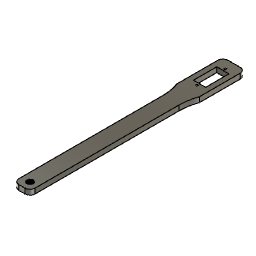
SOAR_Arm_Long-v2 (Autodesk Fusion 360 design; units mm, degrees)
Autodesk Fusion 360 part; units mm, degrees
sketch "Sketch1" plane through (0, 0, 0) normal (0, 0, 1) x (1, 0, 0)
  line L0 (0, 0) -> (16, 0)
  line L1 (16, 0) -> (16, 16)
  line L2 (16, 16) -> (0, 16)
  line L3 (0, 16) -> (0, 0)
  circle A0 centre (8, 8) radius 3.03
  circle A1 centre (8, 8) radius 1.5
  dimension "d1" = 16
  dimension "d2" = 16
  dimension "d3" = 6.06
  dimension "d30" = 3
  constraint horizontal L0
  constraint vertical L1
  constraint horizontal L2
  constraint vertical L3
  constraint coincident L0.start L3.end
  constraint concentric A0 A1
  measures "d1" distance of L0.start L0.end
  measures "d2" distance of L0.start L2.end
  measures "d3" diameter of A0
  measures "d30" diameter of A1
sketch "Sketch2" plane through (0, 0, 0) normal (0, 0, 1) x (1, 0, 0)
  line L0 (0, 21) -> (16, 21)
  line L1 (16, 21) -> (16, 158.5)
  line L2 (16, 158.5) -> (0, 158.5)
  line L3 (0, 158.5) -> (0, 21)
  line L4 (0, 16) -> (16, 16)
  line L5 (16, 16) -> (16, 21)
  line L6 (16, 21) -> (0, 21)
  line L7 (0, 21) -> (0, 16)
  line L8 (0, 158.5) -> (16, 158.5)
  line L9 (16, 158.5) -> (16, 163.5)
  line L10 (16, 163.5) -> (0, 163.5)
  line L11 (0, 163.5) -> (0, 158.5)
  dimension "d17" = 16
  dimension "d18" = 137.5
  constraint horizontal L0
  constraint vertical L1
  constraint horizontal L2
  constraint vertical L3
  constraint horizontal L4
  constraint vertical L5
  constraint horizontal L6
  constraint vertical L7
  constraint horizontal L8
  constraint vertical L9
  constraint horizontal L10
  constraint vertical L11
  measures "d17" distance of L0.start L0.end
  measures "d18" distance of L0.start L2.end
sketch "Sketch3" plane through (0, 0, 0) normal (0, 0, 1) x (1, 0, 0)
  line L0 (-3, 163.5) -> (19, 163.5)
  line L1 (19, 163.5) -> (19, 208.5)
  line L2 (19, 208.5) -> (-3, 208.5)
  line L3 (-3, 208.5) -> (-3, 163.5)
  line L4 (2, 202.25) -> (14, 202.25)
  line L5 (14, 202.25) -> (14, 169.75)
  line L6 (14, 169.75) -> (2, 169.75)
  line L7 (2, 169.75) -> (2, 202.25)
  line L8 (2, 202.25) -> (14, 202.25)
  line L9 (14, 202.25) -> (14, 197.45)
  line L10 (14, 197.45) -> (2, 197.45)
  line L11 (2, 197.45) -> (2, 202.25)
  line L12 (2, 169.75) -> (14, 169.75)
  line L13 (14, 169.75) -> (14, 174.55)
  line L14 (14, 174.55) -> (2, 174.55)
  line L15 (2, 174.55) -> (2, 169.75)
  circle A0 centre (8, 199.85) radius 1
  circle A1 centre (8, 172.15) radius 1
  circle A2 centre (8, 199.85) radius 1.5
  circle A3 centre (8, 172.15) radius 1.5
  dimension "d6" = 45
  dimension "d7" = 12
  dimension "d8" = 32.5
  dimension "d9" = 4.8
  dimension "d44" = 3
  dimension "d45" = 3
  constraint horizontal L0
  constraint vertical L1
  constraint horizontal L2
  constraint vertical L3
  constraint horizontal L4
  constraint vertical L5
  constraint horizontal L6
  constraint vertical L7
  constraint horizontal L8
  constraint vertical L9
  constraint horizontal L10
  constraint vertical L11
  constraint horizontal L12
  constraint vertical L13
  constraint horizontal L14
  constraint vertical L15
  constraint concentric A0 A2
  constraint concentric A1 A3
  measures "d6" distance of L0.start L2.end
  measures "d7" distance of L4.start L4.end
  measures "d8" distance of L4.start L6.end
  measures "d9" distance of L4.start L10.end
  measures "d44" diameter of A2
  measures "d45" diameter of A3
extrude "Extrude1" add sketch "Sketch3" sketch "Sketch2" along normal blind 5 contours L0 L1 L2 L3 | L4 L5 L7 L8 L9 L10 L11 | L5 L6 L7 L12 L13 L14 L15 | A2 | A3 of sketch 2 contours L2 L8 L9 L10 L11 makes body 1
extrude "Extrude3" add sketch "Sketch2" along normal blind 5 contours L0 L1 L2 L3 L6 L8 bodies 1
extrude "Extrude4" add sketch "Sketch1" sketch "Sketch2" along normal blind 5 contours L0 L1 L2 L3 of sketch 2 contours L0 L4 L5 L6 L7 bodies 1
extrude "Extrude5" add sketch "Sketch1" along normal blind 0.5 contours A0 bodies 1
fillet "Fillet1" radius 50 2 edges at (0, 163.5, 2.5) (16, 163.5, 2.5) on bodies 1
sketch "Sketch4" plane through (0, 0, 0) normal (0, 0, 1) x (1, 0, 0)
  line L0 (22.4324, 10.8264) -> (22.3359, 10.6944)
  line L1 (22.5324, 10.9633) -> (22.4324, 10.8264)
  line L2 (22.3359, 10.6944) -> (22.1891, 10.7664)
  line L3 (22.1891, 10.7664) -> (22.0369, 10.8412)
  line L4 (21.8368, 10.7653) -> (21.7725, 10.6084)
  arc A0 (22.0369, 10.8412) -> (21.8368, 10.7653) centre (23, 8) ccw
  arc A1 (22.7448, 10.9891) -> (22.5324, 10.9633) centre (23, 8) ccw
  line L5 (21.7725, 10.6084) -> (21.7104, 10.4571)
  line L6 (21.7104, 10.4571) -> (21.5506, 10.492)
  line L7 (21.5506, 10.492) -> (21.3849, 10.5281)
  arc A2 (21.3849, 10.5281) -> (21.2089, 10.4066) centre (23, 8) ccw
  line L8 (22.8747, 10.8801) -> (23, 10.775)
  line L9 (23, 10.775) -> (23.1253, 10.8801)
  line L10 (23.6641, 10.6944) -> (23.5676, 10.8264)
  line L11 (23.8109, 10.7664) -> (23.6641, 10.6944)
  line L12 (24.2896, 10.4571) -> (24.2275, 10.6084)
  line L13 (24.4494, 10.492) -> (24.2896, 10.4571)
  line L14 (24.8402, 10.0771) -> (24.8161, 10.2389)
  line L15 (25.0036, 10.0727) -> (24.8402, 10.0771)
  line L16 (25.2838, 9.5764) -> (25.2991, 9.7392)
  line L17 (25.4415, 9.533) -> (25.2838, 9.5764)
  line L18 (25.5947, 8.984) -> (25.6485, 9.1384)
  line L19 (25.7374, 8.9042) -> (25.5947, 8.984)
  line L20 (25.7548, 8.3345) -> (25.844, 8.4715)
  line L21 (25.8742, 8.2228) -> (25.7548, 8.3345)
  line L22 (25.7548, 7.6655) -> (25.8742, 7.7772)
  line L23 (25.844, 7.5285) -> (25.7548, 7.6655)
  line L24 (25.5947, 7.016) -> (25.7374, 7.0958)
  line L25 (25.6485, 6.8616) -> (25.5947, 7.016)
  line L26 (25.2838, 6.4236) -> (25.4415, 6.467)
  line L27 (25.2991, 6.2608) -> (25.2838, 6.4236)
  line L28 (24.8402, 5.9229) -> (25.0036, 5.9273)
  line L29 (24.8161, 5.7611) -> (24.8402, 5.9229)
  line L30 (24.2896, 5.5429) -> (24.4494, 5.508)
  line L31 (24.2275, 5.3916) -> (24.2896, 5.5429)
  line L32 (23.6641, 5.3056) -> (23.8109, 5.2336)
  line L33 (23.5676, 5.1736) -> (23.6641, 5.3056)
  line L34 (23, 5.225) -> (23.1253, 5.1199)
  line L35 (22.8747, 5.1199) -> (23, 5.225)
  line L36 (22.3359, 5.3056) -> (22.4324, 5.1736)
  line L37 (22.1891, 5.2336) -> (22.3359, 5.3056)
  line L38 (21.7104, 5.5429) -> (21.7725, 5.3916)
  line L39 (21.5506, 5.508) -> (21.7104, 5.5429)
  line L40 (21.1598, 5.9229) -> (21.1839, 5.7611)
  line L41 (20.9964, 5.9273) -> (21.1598, 5.9229)
  line L42 (20.7162, 6.4236) -> (20.7009, 6.2608)
  line L43 (20.5585, 6.467) -> (20.7162, 6.4236)
  line L44 (20.4053, 7.016) -> (20.3515, 6.8616)
  line L45 (20.2626, 7.0958) -> (20.4053, 7.016)
  line L46 (20.2452, 7.6655) -> (20.156, 7.5285)
  line L47 (20.1258, 7.7772) -> (20.2452, 7.6655)
  line L48 (20.2452, 8.3345) -> (20.1258, 8.2228)
  line L49 (20.156, 8.4715) -> (20.2452, 8.3345)
  line L50 (20.4053, 8.984) -> (20.2626, 8.9042)
  line L51 (20.3515, 9.1384) -> (20.4053, 8.984)
  line L52 (20.7162, 9.5764) -> (20.5585, 9.533)
  line L53 (20.7009, 9.7392) -> (20.7162, 9.5764)
  line L54 (21.1598, 10.0771) -> (20.9964, 10.0727)
  line L55 (21.1839, 10.2389) -> (21.1598, 10.0771)
  line L56 (22.7448, 10.9891) -> (22.8747, 10.8801)
  line L57 (21.2089, 10.4066) -> (21.1839, 10.2389)
  line L58 (20.9964, 10.0727) -> (20.8268, 10.0682)
  line L59 (20.685, 9.908) -> (20.7009, 9.7392)
  arc A3 (20.8268, 10.0682) -> (20.685, 9.908) centre (23, 8) ccw
  line L60 (20.5585, 9.533) -> (20.395, 9.488)
  line L61 (20.2956, 9.2986) -> (20.3515, 9.1384)
  arc A4 (20.395, 9.488) -> (20.2956, 9.2986) centre (23, 8) ccw
  line L62 (20.2626, 8.9042) -> (20.1146, 8.8214)
  arc A5 (20.1146, 8.8214) -> (20.0634, 8.6136) centre (23, 8) ccw
  line L63 (20.0634, 8.6136) -> (20.156, 8.4715)
  line L64 (20.1258, 8.2228) -> (20.0019, 8.107)
  line L65 (20.0019, 7.893) -> (20.1258, 7.7772)
  arc A6 (20.0019, 8.107) -> (20.0019, 7.893) centre (23, 8) ccw
  line L66 (20.156, 7.5285) -> (20.0634, 7.3864)
  line L67 (20.1146, 7.1786) -> (20.2626, 7.0958)
  arc A7 (20.0634, 7.3864) -> (20.1146, 7.1786) centre (23, 8) ccw
  line L68 (20.3515, 6.8616) -> (20.2956, 6.7014)
  arc A8 (20.2956, 6.7014) -> (20.395, 6.512) centre (23, 8) ccw
  line L69 (20.395, 6.512) -> (20.5585, 6.467)
  line L70 (20.7009, 6.2608) -> (20.685, 6.092)
  line L71 (20.8268, 5.9318) -> (20.9964, 5.9273)
  arc A9 (20.685, 6.092) -> (20.8268, 5.9318) centre (23, 8) ccw
  line L72 (21.1839, 5.7611) -> (21.2089, 5.5934)
  line L73 (21.3849, 5.4719) -> (21.5506, 5.508)
  arc A10 (21.2089, 5.5934) -> (21.3849, 5.4719) centre (23, 8) ccw
  line L74 (21.7725, 5.3916) -> (21.8368, 5.2347)
  arc A11 (21.8368, 5.2347) -> (22.0369, 5.1588) centre (23, 8) ccw
  line L75 (22.0369, 5.1588) -> (22.1891, 5.2336)
  line L76 (22.4324, 5.1736) -> (22.5324, 5.0367)
  line L77 (22.7448, 5.0109) -> (22.8747, 5.1199)
  arc A12 (22.5324, 5.0367) -> (22.7448, 5.0109) centre (23, 8) ccw
  line L78 (23.1253, 5.1199) -> (23.2552, 5.0109)
  line L79 (23.4676, 5.0367) -> (23.5676, 5.1736)
  arc A13 (23.2552, 5.0109) -> (23.4676, 5.0367) centre (23, 8) ccw
  line L80 (23.8109, 5.2336) -> (23.9631, 5.1588)
  arc A14 (23.9631, 5.1588) -> (24.1632, 5.2347) centre (23, 8) ccw
  line L81 (24.1632, 5.2347) -> (24.2275, 5.3916)
  line L82 (24.4494, 5.508) -> (24.6151, 5.4719)
  line L83 (24.7911, 5.5934) -> (24.8161, 5.7611)
  arc A15 (24.6151, 5.4719) -> (24.7911, 5.5934) centre (23, 8) ccw
  line L84 (25.0036, 5.9273) -> (25.1732, 5.9318)
  line L85 (25.315, 6.092) -> (25.2991, 6.2608)
  arc A16 (25.1732, 5.9318) -> (25.315, 6.092) centre (23, 8) ccw
  line L86 (25.4415, 6.467) -> (25.605, 6.512)
  arc A17 (25.605, 6.512) -> (25.7044, 6.7014) centre (23, 8) ccw
  line L87 (25.7044, 6.7014) -> (25.6485, 6.8616)
  line L88 (25.7374, 7.0958) -> (25.8854, 7.1786)
  line L89 (25.9366, 7.3864) -> (25.844, 7.5285)
  arc A18 (25.8854, 7.1786) -> (25.9366, 7.3864) centre (23, 8) ccw
  line L90 (25.8742, 7.7772) -> (25.9981, 7.893)
  line L91 (25.9981, 8.107) -> (25.8742, 8.2228)
  arc A19 (25.9981, 7.893) -> (25.9981, 8.107) centre (23, 8) ccw
  line L92 (25.844, 8.4715) -> (25.9366, 8.6136)
  arc A20 (25.9366, 8.6136) -> (25.8854, 8.8214) centre (23, 8) ccw
  line L93 (25.8854, 8.8214) -> (25.7374, 8.9042)
  line L94 (25.6485, 9.1384) -> (25.7044, 9.2986)
  line L95 (25.605, 9.488) -> (25.4415, 9.533)
  arc A21 (25.7044, 9.2986) -> (25.605, 9.488) centre (23, 8) ccw
  line L96 (25.2991, 9.7392) -> (25.315, 9.908)
  line L97 (25.1732, 10.0682) -> (25.0036, 10.0727)
  arc A22 (25.315, 9.908) -> (25.1732, 10.0682) centre (23, 8) ccw
  line L98 (24.8161, 10.2389) -> (24.7911, 10.4066)
  arc A23 (24.7911, 10.4066) -> (24.6151, 10.5281) centre (23, 8) ccw
  line L99 (24.6151, 10.5281) -> (24.4494, 10.492)
  line L100 (24.2275, 10.6084) -> (24.1632, 10.7653)
  line L101 (23.9631, 10.8412) -> (23.8109, 10.7664)
  arc A24 (24.1632, 10.7653) -> (23.9631, 10.8412) centre (23, 8) ccw
  line L102 (23.5676, 10.8264) -> (23.4676, 10.9633)
  line L103 (23.1253, 10.8801) -> (23.2552, 10.9891)
  arc A25 (23.4676, 10.9633) -> (23.2552, 10.9891) centre (23, 8) ccw
  circle A26 centre (23, 8) radius 3.1
  dimension "d41" = 6.2
  constraint concentric A0 A26
  measures "d41" diameter of A26
extrude "Extrude6" add sketch "Sketch4" along normal blind 4.5 separate body makes body 2
scale "Scale1" factor 1.02 about (19.9, 8, 4.5) bodies 2
move_body "Move3" bodies 2 to x (1, 0, 0) y (0, 1, 0) z (0, 0, 1) at (-15.06, -0.06, 0.5)
combine "Combine1" operation add target body 1 tool bodies 2
fillet "Fillet2" radius 5 4 edges at (-3, 208.5, 2.5) (19, 208.5, 2.5) (16, 0, 2.5) (0, 0, 2.5) on bodies 1
named bodies: "Body1", "Body4"
